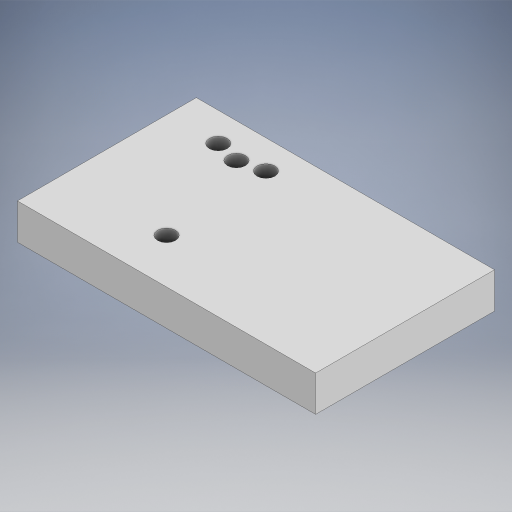
# Autodesk Inventor part: Seitenwand
Saved by Autodesk Inventor 2024 (Build 280153000, 153)
## iProperties
Created: 2023-08-24
Part Number: Seitenwand
Material: Generisch
Document SubType Name: Modeling
Designer: rapp
Density: 1 g/cm^3
Appearance: Vorgabe
Author: rapp
Autodesk Inventor part; units mm, degrees
ref_plane "YZ Plane" through (0, 0, 0) normal (1, 0, 0) x (0, 1, 0)
ref_plane "XZ Plane" through (0, 0, 0) normal (0, 1, 0) x (-1, 0, 0)
ref_plane "XY Plane" through (0, 0, 0) normal (0, 0, 1) x (1, 0, 0)
sketch "Skizze1" plane through (0, 0, 0) normal (0, 0, 1) x (1, 0, 0)
  line L0 (0, 0) -> (100, 0)
  line L1 (100, 0) -> (100, 60)
  line L2 (100, 60) -> (0, 60)
  line L3 (0, 60) -> (0, 0)
  dimension "d0" = 100
  dimension "d1" = 60
  constraints: 8 end point, 2 parallel, 1 horizontal, 1 perpendicular
  measures "d0" distance of L2.end L1.end
  measures "d1" distance of L1.end L0.end
extrude "Extrusion1" add sketch "Skizze1" along normal blind 12
sketch "Skizze2" plane through (0, 0, 12) normal (0, 0, 1) x (1, 0, 0)
  circle A0 centre (33, 50.3439) radius 3
  circle A1 centre (17, 50.3439) radius 3
  point P0 (0, 0)
  point P1 (25, 45.3439)
  constraints: 2 centre point, 2 coincident, 5 other
hole "Bohrung1" at (17, 50.3439, 12) at (33, 50.3439, 12) direction (0, 0, -1) diameter 6 end through all
sketch "Skizze4" plane through (0, 0, 12) normal (0, 0, 1) x (1, 0, 0)
  circle A0 centre (25, 48.4439) radius 3.1
  point P0 (0, 0)
  point P1 (25, 45.3439)
  constraints: 1 coincident, 1 vertical alignment, 3 other
hole "Bohrung3" at (25, 48.4439, 12) direction (0, 0, -1) diameter 6 end through all
sketch "Skizze6" plane through (0, 0, 0) normal (0, 0, -1) x (-1, 0, 0)
  circle A0 centre (-35, 15) radius 2.5
  point P0 (0, 0)
  constraints: 1 centre point, 1 coincident, 2 other
hole "Bohrung5" at (35, 15, 0) direction (0, 0, 1) diameter 6 end through all
